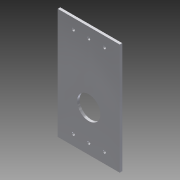
# Autodesk Inventor part: bearingplate(bp)
Saved by Autodesk Inventor 2015 (Build 190159000, 159)
## iProperties
Created: 2015-10-02
Part Number: bearingplate(bp)
Material: Aluminum 6061
Document SubType Name: Sheet Metal
Designer: elilitwack
Density: 2.7 g/cm^3
Sheet Metal Rule: Default
Appearance: Aluminum - Flat
Mass: 120.566 g
Surface Area: 317.438 cm^2
Volume: 44.6539 cm^3
Author: elilitwack
Autodesk Inventor part; units mm, degrees
ref_plane "YZ Plane" through (0, 0, 0) normal (1, 0, 0) x (0, 1, 0)
ref_plane "XZ Plane" through (0, 0, 0) normal (0, 1, 0) x (-1, 0, 0)
ref_plane "XY Plane" through (0, 0, 0) normal (0, 0, 1) x (1, 0, 0)
sketch "face_sketch" plane through (0, 0, 0) normal (0, 0, 1) x (1, 0, 0)
  line L0 (0, 0) -> (76.2, 0)
  line L1 (76.2, 0) -> (76.2, 136.5504)
  line L2 (76.2, 136.5504) -> (0, 136.5504)
  line L3 (0, 136.5504) -> (0, 0)
  dimension "d0" = 136.5504
  dimension "d1" = 76.2
  constraints: 8 end point, 2 parallel, 1 horizontal, 1 perpendicular
  measures "d0" distance of L0.end L1.end
  measures "d1" distance of L1.end L2.end
extrude "Plate1" add sketch "face_sketch" along normal blind 3.048
sketch "rivet_holes_sketch" plane through (0, 0, 3.048) normal (0, 0, 1) x (1, 0, 0)
  line L0 (0, 0) -> (0, 136.5504) projected
  line L1 (76.2, 136.5504) -> (76.2, 0) projected
  line L2 (76.2, 0) -> (76.2, 136.5504) construction
  line L3 (57.15, 123.8504) -> (38.1, 123.8504) construction
  line L4 (38.1, 123.8504) -> (19.05, 123.8504) construction
  line L5 (19.05, 123.8504) -> (0, 123.8504) construction
  line L6 (0, 136.5504) -> (0, 0) construction
  line L7 (0, 136.5504) -> (76.2, 136.5504) construction
  line L8 (38.1, 136.5504) -> (38.1, 68.2752) construction
  line L9 (38.1, 68.2752) -> (38.1, 0) construction
  line L10 (0, 0) -> (76.2, 0) construction
  line L11 (38.1, 68.2752) -> (0, 68.2752) construction
  line L12 (38.1, 68.2752) -> (76.2, 68.2752) construction
  line L13 (38.1, 68.2752) -> (38.1, 136.5504) construction
  line L14 (57.15, 123.8504) -> (76.2, 123.8504) construction
  point P0 (19.05, 12.7)
  point P1 (38.1, 12.7)
  point P2 (57.15, 12.7)
  dimension "gb_bearing_diameter" = 28.575
  dimension "d3" = 19.05
  dimension "d4" = 19.05
  dimension "d5" = 19.05
  dimension "d42" = 12.7
  dimension "d43" = 19.05
  constraints: 18 end point, 4 midpoint, 3 point on line, 3 symmetric about line, 1 collinear, 1 perpendicular, 1 vertical
  measures "d3" distance from line of L0 L4.end
  measures "d4" distance of L3.end L4.end
  measures "d5" distance of L3.start L3.end
  measures "d42" distance between parallel lines of L7 L4
  measures "d43" distance of L3.start L14.end
hole "rivet_holes" at (19.05, 123.8504, 3.048) at (38.1, 123.8504, 3.048) at (57.15, 123.8504, 3.048) at (19.05, 12.7, 3.048) at (38.1, 12.7, 3.048) at (57.15, 12.7, 3.048) direction (0, 0, -1) diameter 3.5719 depth 3.048 tip angle 118
sketch "bearing_hole_sketch" plane through (0, 0, 3.048) normal (0, 0, 1) x (1, 0, 0)
  line L0 (0, 136.5504) -> (0, 0) projected
  line L1 (0, 45.1612) -> (38.1, 45.1612) construction
  line L2 (76.2, 0) -> (76.2, 136.5504) projected
  line L3 (76.2, 0) -> (0, 0) projected
  line L4 (38.1, 45.1612) -> (76.2, 45.1612) construction
  dimension "d18" = 45.1612
  constraints: 4 end point, 2 horizontal, 2 point on line, 1 coincident, 1 collinear
  measures "d18" distance between parallel lines of L3 L1
hole "bearing_hole" at (38.1, 45.1612, 3.048) direction (0, 0, -1) diameter 28.575 depth 3.048 tip angle 118
equation "\"gb_bearing_diameter\" = 28.575"
equation "\"d3\" = st_rivet_distance"
equation "\"d4\" = st_rivet_distance"
equation "\"d5\" = st_rivet_distance"
equation "\"d42\" = 0.5 * st_outer_diameter"
equation "\"d43\" = st_rivet_distance"
equation "\"d10\" = rv_hole_diameter"
equation "\"d15\" = Thickness"
equation "\"d19\" = gb_bearing_diameter"
equation "\"d24\" = Thickness"
equation "\"d0\" = bp_height"
equation "\"d1\" = bp_width"
equation "\"Thickness\" = bp_thickness"
equation "\"BendRadius\" = Thickness"
equation "\"BendReliefWidth\" = Thickness"
equation "\"BendReliefDepth\" = 0.5 * Thickness"
equation "\"CornerReliefSize\" = 4 * Thickness"
equation "\"MinimumRemnant\" = 2 * Thickness"
equation "\"TransitionRadius\" = BendRadius"
equation "\"JacobiRadiusSize\" = BendRadius"
equation "\"GapSize\" = Thickness"
equation "\"st_outer_diameter\" = 25.4"
equation "\"st_wall_thickness\" = 1.5875"
equation "\"st_length\" = 685.8"
equation "\"st_gbmh_from_center\" = 0.5 * gb_mh_seperation"
equation "\"st_cutout_depth\" = 254"
equation "\"st_rivet_distance\" = 19.05"
equation "\"rv_hole_diameter\" = 3.57187"
equation "\"gb_mh_seperation\" = 111.1504"
equation "\"gb_mh_diameter\" = 6.35"
equation "\"bp_thickness\" = 3.048"
equation "\"bp_height\" = gb_mh_seperation + st_outer_diameter"
equation "\"bp_width\" = 4 * st_rivet_distance"
equation "\"d2\" = BendRadius"
equation "\"st_cutout_depth_left\" = 203.2"
equation "\"st_cutout_depth_right\" = 203.2"
equation "\"gb_width\" = 127"
equation "\"gb_axle_from_edge\" = 38.1"
equation "\"magic_offset\" = 3.175"
equation "\"magic_axle_offset\" = 2.286"
equation "\"bp_axle_height\" = magic_axle_offset + gb_axle_from_edge + gb_to_bottom_of_side_assembly"
equation "\"gb_to_bottom_of_side_assembly\" = 4.7752"
equation "\"bp_tensioner_width\" = 6.35"
equation "\"bp_tensioner_height\" = 50.8"
equation "\"bp_tensioner_from_top\" = 38.1"
equation "\"bp_tensioner_from_bottom\" = 38.1"
equation "\"bp_tensioner_from_side\" = 25.4"
equation "\"bp_tensioner_wood_mount_diameter\" = 6.35"
equation "\"bp_tensioner_wood_mount_from_tensioner_top\" = 12.7"
equation "\"twb_width\" = st_outer_diameter"
equation "\"twb_length\" = bp_tensioner_width + 2 * twb_margin_on_each_side"
equation "\"twb_height\" = 2 * bp_tensioner_wood_mount_diameter + bp_tensioner_height + 2 * bp_tensioner_wood_mount_from_tensioner_top + twb_margin_on_each_side"
equation "\"twb_margin_on_each_side\" = 6.35"
equation "\"twb_tensioner_from_edge\" = -0.5 * bp_tensioner_height + 0.5 * twb_height"
equation "\"gb_mh_seperation_alt\" = 111.125"
equation "\"gb_axle_from_edge_alt\" = 43.1546"
equation "\"bp_axle_height_alt\" = magic_axle_offset + gb_axle_from_edge_alt + gb_to_bottom_of_side_assembly"
body "Solid1"
